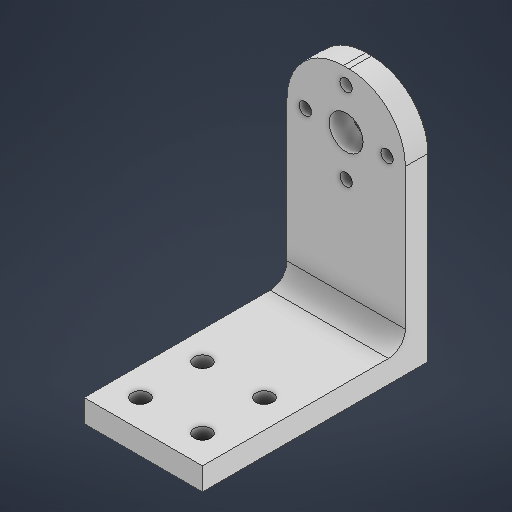
# Autodesk Inventor part: L1
Saved by Autodesk Inventor 2026.1 (Build 301233000, 233)
## iProperties
Created: 2025-09-17
Part Number: L1
Material: Generic
Document SubType Name: Modeling
Designer: emanuel
Density: 1 g/cm^3
Appearance: Default
Author: emanuel
Autodesk Inventor part; units mm, degrees
ref_plane "YZ Plane" through (0, 0, 0) normal (1, 0, 0) x (0, 1, 0)
ref_plane "XZ Plane" through (0, 0, 0) normal (0, 1, 0) x (-1, 0, 0)
ref_plane "XY Plane" through (0, 0, 0) normal (0, 0, 1) x (1, 0, 0)
sketch "Sketch1" plane through (0, 0, 0) normal (1, 0, 0) x (0, 1, 0)
  line L0 (0, 0) -> (0, -36)
  line L1 (0, -36) -> (38, -36)
  line L2 (0, 0) -> (-4, 0)
  line L3 (-4, 0) -> (-4, -40)
  line L4 (-4, -40) -> (38, -40)
  line L5 (38, -40) -> (38, -36)
  dimension "d0" = 36
  dimension "d1" = 38
  dimension "d2" = 4
  dimension "d3" = 40
  constraints: 12 end point, 4 perpendicular, 1 horizontal, 1 vertical
  measures "d0" distance of L0.start L0.end
  measures "d1" distance of L0.end L1.end
  measures "d2" distance of L0.start L2.end
  measures "d3" distance of L2.end L3.end
extrude "Extrusion1" add sketch "Sketch1" along normal blind 21
fillet "Fillet1" radius 10 2 edges at (21, 38, -38) (0, 38, -38)
sketch "Sketch2" plane through (0, 0, -36) normal (0, 0, 1) x (1, 0, 0)
  arc A0 (10, 38) -> (0, 28) centre (10, 28) ccw projected
  line L0 (0, 28) -> (21, 28)
  line L1 (0, 28) -> (0, 0) projected
  line L2 (0, 28) -> (10.5, 28)
  circle A1 centre (10.5, 28) radius 8
  circle A2 centre (10.5, 28) radius 6.5
  line L3 (4, 28) -> (2.5, 28)
  circle A3 centre (3.25, 28) radius 1.1
  line L4 (17, 28) -> (18.5, 28)
  circle A4 centre (17.75, 28) radius 1.1
  line L5 (10.5, 28) -> (10.5, 36)
  line L6 (10.5, 28) -> (10.5, 20)
  line L7 (10.5, 36) -> (10.5, 34.5)
  line L8 (10.5, 20) -> (10.5, 21.5)
  circle A5 centre (10.5, 35.25) radius 1.1
  circle A6 centre (10.5, 20.75) radius 1.1
  circle A7 centre (10.5, 28) radius 3
  dimension "d7" = 10.5
  dimension "d8" = 16
  dimension "d9" = 13
  dimension "d10" = 2.2
  dimension "d11" = 2.2
  dimension "d12" = 2.2
  dimension "d13" = 2.2
  dimension "d14" = 6
  constraints: 16 end point, 8 point on circle, 7 centre point, 7 point on line, 5 midpoint, 3 coincident, 1 vertical
  measures "d7" distance of L0.start L2.end
  measures "d8" diameter of A1
  measures "d9" diameter of A2
  measures "d10" diameter of A3
  measures "d11" diameter of A4
  measures "d12" diameter of A5
  measures "d13" diameter of A6
  measures "d14" diameter of A7
extrude "Extrusion2" cut sketch "Sketch2" against normal blind 21 contours A2 A3 A1 L0 | A2 A3 L0 | L0 A1 A3 A2 | L0 A3 A2 | A1 A3 L0 | L0 A3 A1 | A7 L5 L0 | L0 L6 A7 | A5 A1 L5 A2 | A2 L5 A5 | A6 L6 A2 | A2 L6 A1 A6 | A5 A1 | A1 A6 | L5 A7 L0 | L0 A7 L6 | L5 A1 A5 A2 | A2 A5 L5 | L6 A6 A2 | A2 A6 A1 L6 | A4 L0 A1 | A1 L0 A2 A4 | A4 A2 L0 A1 | A1 L0 A4 | A4 A2 L0 | L0 A2 A4
sketch "Sketch3" plane through (0, 0, 0) normal (0, 1, 0) x (1, 0, 0)
  line L0 (0, 36) -> (0, 0) projected
  line L1 (0, 0) -> (5, 0)
  line L2 (5, 0) -> (5, 5)
  line L3 (5, 5) -> (0, 5)
  line L4 (0, 5) -> (0, 0)
  line L5 (5, 5) -> (16, 5)
  line L6 (16, 5) -> (16, 16)
  line L7 (16, 16) -> (5, 16)
  line L8 (5, 16) -> (5, 5)
  circle A0 centre (5, 5) radius 1.5
  circle A1 centre (5, 16) radius 1.5
  circle A2 centre (16, 5) radius 1.5
  circle A3 centre (16, 16) radius 1.5
  dimension "d17" = 5
  dimension "d18" = 5
  dimension "d19" = 11
  dimension "d20" = 11
  dimension "d21" = 3
  dimension "d22" = 3
  dimension "d23" = 3
  dimension "d24" = 3
  constraints: 16 end point, 4 centre point, 4 coincident, 4 parallel, 2 horizontal, 2 perpendicular
  measures "d17" distance of L3.end L2.end
  measures "d18" distance of L2.end L1.end
  measures "d19" distance of L7.end L6.end
  measures "d20" distance of L6.end L5.end
  measures "d21" diameter of A0
  measures "d22" diameter of A1
  measures "d23" diameter of A2
  measures "d24" diameter of A3
extrude "Extrusion3" cut sketch "Sketch3" against normal blind 21 contours A0 L8 L3 | L3 L2 A0 | L5 A0 L2 | L8 A0 L5 | A1 L7 L8 | L8 L7 A1 | A2 L6 L5 | L5 L6 A2 | A3 L6 L7 | L7 L6 A3
fillet "Fillet2" radius 3 1 edges at (10.5, 0, -36)
body "Solid1"
